Autodesk Inventor part; units mm, degrees
(part 2 of 2)
  circle A612 centre (-1.45, 4) radius 0.5
  circle A613 centre (1.1, 4) radius 0.5
  circle A614 centre (3.65, 4) radius 0.5
  circle A615 centre (6.2, 4) radius 0.5
  circle A616 centre (8.75, 4) radius 0.5
  circle A617 centre (11.3, 4) radius 0.5
  circle A618 centre (13.85, 4) radius 0.5
  circle A619 centre (16.4, 4) radius 0.5
  circle A620 centre (18.95, 4) radius 0.5
  circle A621 centre (21.5, 4) radius 0.5
  circle A622 centre (24.05, 4) radius 0.5
  circle A623 centre (26.6, 4) radius 0.5
  circle A624 centre (29.15, 4) radius 0.5
  circle A625 centre (-29.5, 1.5) radius 0.5
  circle A626 centre (-26.95, 1.5) radius 0.5
  circle A627 centre (-24.4, 1.5) radius 0.5
  circle A628 centre (-21.85, 1.5) radius 0.5
  circle A629 centre (-19.3, 1.5) radius 0.5
  circle A630 centre (-16.75, 1.5) radius 0.5
  circle A631 centre (-14.2, 1.5) radius 0.5
  circle A632 centre (-11.65, 1.5) radius 0.5
  circle A633 centre (-9.1, 1.5) radius 0.5
  circle A634 centre (-6.55, 1.5) radius 0.5
  circle A635 centre (-4, 1.5) radius 0.5
  circle A636 centre (-1.45, 1.5) radius 0.5
  circle A637 centre (1.1, 1.5) radius 0.5
  circle A638 centre (3.65, 1.5) radius 0.5
  circle A639 centre (6.2, 1.5) radius 0.5
  circle A640 centre (8.75, 1.5) radius 0.5
  circle A641 centre (11.3, 1.5) radius 0.5
  circle A642 centre (13.85, 1.5) radius 0.5
  circle A643 centre (16.4, 1.5) radius 0.5
  circle A644 centre (18.95, 1.5) radius 0.5
  circle A645 centre (21.5, 1.5) radius 0.5
  circle A646 centre (24.05, 1.5) radius 0.5
  circle A647 centre (26.6, 1.5) radius 0.5
  circle A648 centre (29.15, 1.5) radius 0.5
  circle A649 centre (-29.5, -1) radius 0.5
  circle A650 centre (-26.95, -1) radius 0.5
  circle A651 centre (-24.4, -1) radius 0.5
  circle A652 centre (-21.85, -1) radius 0.5
  circle A653 centre (-19.3, -1) radius 0.5
  circle A654 centre (-16.75, -1) radius 0.5
  circle A655 centre (-14.2, -1) radius 0.5
  circle A656 centre (-11.65, -1) radius 0.5
  circle A657 centre (-9.1, -1) radius 0.5
  circle A658 centre (-6.55, -1) radius 0.5
  circle A659 centre (-4, -1) radius 0.5
  circle A660 centre (-1.45, -1) radius 0.5
  circle A661 centre (1.1, -1) radius 0.5
  circle A662 centre (3.65, -1) radius 0.5
  circle A663 centre (6.2, -1) radius 0.5
  circle A664 centre (8.75, -1) radius 0.5
  circle A665 centre (11.3, -1) radius 0.5
  circle A666 centre (13.85, -1) radius 0.5
  circle A667 centre (16.4, -1) radius 0.5
  circle A668 centre (18.95, -1) radius 0.5
  circle A669 centre (21.5, -1) radius 0.5
  circle A670 centre (24.05, -1) radius 0.5
  circle A671 centre (26.6, -1) radius 0.5
  circle A672 centre (29.15, -1) radius 0.5
  circle A673 centre (-29.5, -3.5) radius 0.5
  circle A674 centre (-26.95, -3.5) radius 0.5
  circle A675 centre (-24.4, -3.5) radius 0.5
  circle A676 centre (-21.85, -3.5) radius 0.5
  circle A677 centre (-19.3, -3.5) radius 0.5
  circle A678 centre (-16.75, -3.5) radius 0.5
  circle A679 centre (-14.2, -3.5) radius 0.5
  circle A680 centre (-11.65, -3.5) radius 0.5
  circle A681 centre (-9.1, -3.5) radius 0.5
  circle A682 centre (-6.55, -3.5) radius 0.5
  circle A683 centre (-4, -3.5) radius 0.5
  circle A684 centre (-1.45, -3.5) radius 0.5
  circle A685 centre (1.1, -3.5) radius 0.5
  circle A686 centre (3.65, -3.5) radius 0.5
  circle A687 centre (6.2, -3.5) radius 0.5
  circle A688 centre (8.75, -3.5) radius 0.5
  circle A689 centre (11.3, -3.5) radius 0.5
  circle A690 centre (13.85, -3.5) radius 0.5
  circle A691 centre (16.4, -3.5) radius 0.5
  circle A692 centre (18.95, -3.5) radius 0.5
  circle A693 centre (21.5, -3.5) radius 0.5
  circle A694 centre (24.05, -3.5) radius 0.5
  circle A695 centre (26.6, -3.5) radius 0.5
  circle A696 centre (29.15, -3.5) radius 0.5
  circle A697 centre (-29.5, -6) radius 0.5
  circle A698 centre (-26.95, -6) radius 0.5
  circle A699 centre (-24.4, -6) radius 0.5
  circle A700 centre (-21.85, -6) radius 0.5
  circle A701 centre (-19.3, -6) radius 0.5
  circle A702 centre (-16.75, -6) radius 0.5
  circle A703 centre (-14.2, -6) radius 0.5
  circle A704 centre (-11.65, -6) radius 0.5
  circle A705 centre (-9.1, -6) radius 0.5
  circle A706 centre (-6.55, -6) radius 0.5
  circle A707 centre (-4, -6) radius 0.5
  circle A708 centre (-1.45, -6) radius 0.5
  circle A709 centre (1.1, -6) radius 0.5
  circle A710 centre (3.65, -6) radius 0.5
  circle A711 centre (6.2, -6) radius 0.5
  circle A712 centre (8.75, -6) radius 0.5
  circle A713 centre (11.3, -6) radius 0.5
  circle A714 centre (13.85, -6) radius 0.5
  circle A715 centre (16.4, -6) radius 0.5
  circle A716 centre (18.95, -6) radius 0.5
  circle A717 centre (21.5, -6) radius 0.5
  circle A718 centre (24.05, -6) radius 0.5
  circle A719 centre (26.6, -6) radius 0.5
  circle A720 centre (29.15, -6) radius 0.5
  circle A721 centre (-29.5, -8.5) radius 0.5
  circle A722 centre (-26.95, -8.5) radius 0.5
  circle A723 centre (-24.4, -8.5) radius 0.5
  circle A724 centre (-21.85, -8.5) radius 0.5
  circle A725 centre (-19.3, -8.5) radius 0.5
  circle A726 centre (-16.75, -8.5) radius 0.5
  circle A727 centre (-14.2, -8.5) radius 0.5
  circle A728 centre (-11.65, -8.5) radius 0.5
  circle A729 centre (-9.1, -8.5) radius 0.5
  circle A730 centre (-6.55, -8.5) radius 0.5
  circle A731 centre (-4, -8.5) radius 0.5
  circle A732 centre (-1.45, -8.5) radius 0.5
  circle A733 centre (1.1, -8.5) radius 0.5
  circle A734 centre (3.65, -8.5) radius 0.5
  circle A735 centre (6.2, -8.5) radius 0.5
  circle A736 centre (8.75, -8.5) radius 0.5
  circle A737 centre (11.3, -8.5) radius 0.5
  circle A738 centre (13.85, -8.5) radius 0.5
  circle A739 centre (16.4, -8.5) radius 0.5
  circle A740 centre (18.95, -8.5) radius 0.5
  circle A741 centre (21.5, -8.5) radius 0.5
  circle A742 centre (24.05, -8.5) radius 0.5
  circle A743 centre (26.6, -8.5) radius 0.5
  circle A744 centre (29.15, -8.5) radius 0.5
  circle A745 centre (-29.5, -11) radius 0.5
  circle A746 centre (-26.95, -11) radius 0.5
  circle A747 centre (-24.4, -11) radius 0.5
  circle A748 centre (-21.85, -11) radius 0.5
  circle A749 centre (-19.3, -11) radius 0.5
  circle A750 centre (-16.75, -11) radius 0.5
  circle A751 centre (-14.2, -11) radius 0.5
  circle A752 centre (-11.65, -11) radius 0.5
  circle A753 centre (-9.1, -11) radius 0.5
  circle A754 centre (-6.55, -11) radius 0.5
  circle A755 centre (-4, -11) radius 0.5
  circle A756 centre (-1.45, -11) radius 0.5
  circle A757 centre (1.1, -11) radius 0.5
  circle A758 centre (3.65, -11) radius 0.5
  circle A759 centre (6.2, -11) radius 0.5
  circle A760 centre (8.75, -11) radius 0.5
  circle A761 centre (11.3, -11) radius 0.5
  circle A762 centre (13.85, -11) radius 0.5
  circle A763 centre (16.4, -11) radius 0.5
  circle A764 centre (18.95, -11) radius 0.5
  circle A765 centre (21.5, -11) radius 0.5
  circle A766 centre (24.05, -11) radius 0.5
  circle A767 centre (26.6, -11) radius 0.5
  circle A768 centre (29.15, -11) radius 0.5
  circle A769 centre (-29.5, -13.5) radius 0.5
  circle A770 centre (-26.95, -13.5) radius 0.5
  circle A771 centre (-24.4, -13.5) radius 0.5
  circle A772 centre (-21.85, -13.5) radius 0.5
  circle A773 centre (-19.3, -13.5) radius 0.5
  circle A774 centre (-16.75, -13.5) radius 0.5
  circle A775 centre (-14.2, -13.5) radius 0.5
  circle A776 centre (-11.65, -13.5) radius 0.5
  circle A777 centre (-9.1, -13.5) radius 0.5
  circle A778 centre (-6.55, -13.5) radius 0.5
  circle A779 centre (-4, -13.5) radius 0.5
  circle A780 centre (-1.45, -13.5) radius 0.5
  circle A781 centre (1.1, -13.5) radius 0.5
  circle A782 centre (3.65, -13.5) radius 0.5
  circle A783 centre (6.2, -13.5) radius 0.5
  circle A784 centre (8.75, -13.5) radius 0.5
  circle A785 centre (11.3, -13.5) radius 0.5
  circle A786 centre (13.85, -13.5) radius 0.5
  circle A787 centre (16.4, -13.5) radius 0.5
  circle A788 centre (18.95, -13.5) radius 0.5
  circle A789 centre (21.5, -13.5) radius 0.5
  circle A790 centre (24.05, -13.5) radius 0.5
  circle A791 centre (26.6, -13.5) radius 0.5
  circle A792 centre (29.15, -13.5) radius 0.5
  circle A793 centre (-29.5, -16) radius 0.5
  circle A794 centre (-26.95, -16) radius 0.5
  circle A795 centre (-24.4, -16) radius 0.5
  circle A796 centre (-21.85, -16) radius 0.5
  circle A797 centre (-19.3, -16) radius 0.5
  circle A798 centre (-16.75, -16) radius 0.5
  circle A799 centre (-14.2, -16) radius 0.5
  circle A800 centre (-11.65, -16) radius 0.5
  circle A801 centre (-9.1, -16) radius 0.5
  circle A802 centre (-6.55, -16) radius 0.5
  circle A803 centre (-4, -16) radius 0.5
  circle A804 centre (-1.45, -16) radius 0.5
  circle A805 centre (1.1, -16) radius 0.5
  circle A806 centre (3.65, -16) radius 0.5
  circle A807 centre (6.2, -16) radius 0.5
  circle A808 centre (8.75, -16) radius 0.5
  circle A809 centre (11.3, -16) radius 0.5
  circle A810 centre (13.85, -16) radius 0.5
  circle A811 centre (16.4, -16) radius 0.5
  circle A812 centre (18.95, -16) radius 0.5
  circle A813 centre (21.5, -16) radius 0.5
  circle A814 centre (24.05, -16) radius 0.5
  circle A815 centre (26.6, -16) radius 0.5
  circle A816 centre (29.15, -16) radius 0.5
  circle A817 centre (-29.5, -18.5) radius 0.5
  circle A818 centre (-26.95, -18.5) radius 0.5
  circle A819 centre (-24.4, -18.5) radius 0.5
  circle A820 centre (-21.85, -18.5) radius 0.5
  circle A821 centre (-19.3, -18.5) radius 0.5
  circle A822 centre (-16.75, -18.5) radius 0.5
  circle A823 centre (-14.2, -18.5) radius 0.5
  circle A824 centre (-11.65, -18.5) radius 0.5
  circle A825 centre (-9.1, -18.5) radius 0.5
  circle A826 centre (-6.55, -18.5) radius 0.5
  circle A827 centre (-4, -18.5) radius 0.5
  circle A828 centre (-1.45, -18.5) radius 0.5
  circle A829 centre (1.1, -18.5) radius 0.5
  circle A830 centre (3.65, -18.5) radius 0.5
  circle A831 centre (6.2, -18.5) radius 0.5
  circle A832 centre (8.75, -18.5) radius 0.5
  circle A833 centre (11.3, -18.5) radius 0.5
  circle A834 centre (13.85, -18.5) radius 0.5
  circle A835 centre (16.4, -18.5) radius 0.5
  circle A836 centre (18.95, -18.5) radius 0.5
  circle A837 centre (21.5, -18.5) radius 0.5
  circle A838 centre (24.05, -18.5) radius 0.5
  circle A839 centre (26.6, -18.5) radius 0.5
  circle A840 centre (29.15, -18.5) radius 0.5
  circle A841 centre (-29.5, -21) radius 0.5
  circle A842 centre (-26.95, -21) radius 0.5
  circle A843 centre (-24.4, -21) radius 0.5
  circle A844 centre (-21.85, -21) radius 0.5
  circle A845 centre (-19.3, -21) radius 0.5
  circle A846 centre (-16.75, -21) radius 0.5
  circle A847 centre (-14.2, -21) radius 0.5
  circle A848 centre (-11.65, -21) radius 0.5
  circle A849 centre (-9.1, -21) radius 0.5
  circle A850 centre (-6.55, -21) radius 0.5
  circle A851 centre (-4, -21) radius 0.5
  circle A852 centre (-1.45, -21) radius 0.5
  circle A853 centre (1.1, -21) radius 0.5
  circle A854 centre (3.65, -21) radius 0.5
  circle A855 centre (6.2, -21) radius 0.5
  circle A856 centre (8.75, -21) radius 0.5
  circle A857 centre (11.3, -21) radius 0.5
  circle A858 centre (13.85, -21) radius 0.5
  circle A859 centre (16.4, -21) radius 0.5
  circle A860 centre (18.95, -21) radius 0.5
  circle A861 centre (21.5, -21) radius 0.5
  circle A862 centre (24.05, -21) radius 0.5
  circle A863 centre (26.6, -21) radius 0.5
  circle A864 centre (29.15, -21) radius 0.5
  point P0 (0, 0)
  dimension "d33" = 1.75
  dimension "d38" = 2.55
  dimension "d41" = 2.5
  dimension "d46" = 2.55
  dimension "d49" = 2.5
  constraints: 864 centre point, 4 end point, 3 vertical, 2 coincident, 2 horizontal, 1 collinear, 1 concentric, 1724 other
  measures "d33" diameter of A1
  measures "d38" distance of A1.centre A2.centre
  measures "d41" distance of A1.centre A25.centre
  measures "d46" distance of A433.centre A434.centre
  measures "d49" distance of A433.centre A457.centre
extrude "Extrusion7" add sketch "Skizze4" along normal blind 0.05 contours A1
pattern_linear "Rechteckige Anordnung1" count 24 spacing 2.55 along (1, 0, 0) count 18 spacing 2.5 along (0, 0, 1) of "Extrusion7"
